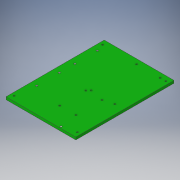
# Autodesk Inventor part: ModBoard-Bottom
Saved by Autodesk Inventor 2018 (Build 220112000, 112)
## iProperties
Created: 2017-12-22
Part Number: ModBoard-Bottom
Material: Generic
Document SubType Name: Modeling
Designer: jklei
Density: 1 g/cm^3
Appearance: Default
Author: jklei
Autodesk Inventor part; units mm, degrees
ref_plane "YZ Plane" through (0, 0, 0) normal (1, 0, 0) x (0, 1, 0)
ref_plane "XZ Plane" through (0, 0, 0) normal (0, 1, 0) x (-1, 0, 0)
ref_plane "XY Plane" through (0, 0, 0) normal (0, 0, 1) x (1, 0, 0)
sketch "Sketch1" plane through (0, 0, 0) normal (0, 1, 0) x (-1, 0, 0)
  line L0 (0, 0) -> (-171.45, 0)
  line L1 (-171.45, 0) -> (-171.45, -241.3)
  line L2 (-171.45, -241.3) -> (0, -241.3)
  line L3 (0, -241.3) -> (0, 0)
  dimension "d0" = 171.45
  dimension "d1" = 241.3
  constraints: 8 end point, 2 parallel, 1 horizontal, 1 perpendicular
  measures "d0" distance of L2.end L1.end
  measures "d1" distance of L1.end L0.end
extrude "Extrusion1" add sketch "Sketch1" along normal blind 6.35
sketch "Sketch2" plane through (0, 6.35, 0) normal (0, 1, 0) x (1, 0, 0)
  line L0 (0, 0) -> (8, 0)
  line L1 (0, 0) -> (171.45, 0) projected
  line L2 (8, 0) -> (8, 12)
  line L3 (171.45, 0) -> (163.45, 0)
  line L4 (163.45, 0) -> (163.45, 12)
  line L5 (171.45, 241.3) -> (0, 241.3) projected
  line L6 (0, 241.3) -> (8, 241.3)
  line L7 (8, 241.3) -> (8, 229.3)
  line L8 (171.45, 241.3) -> (163.45, 241.3)
  line L9 (163.45, 241.3) -> (163.45, 229.3)
  circle A0 centre (8, 229.3) radius 2.1
  circle A1 centre (163.45, 229.3) radius 2.1
  circle A2 centre (163.45, 12) radius 2.1
  circle A3 centre (8, 12) radius 2.1
  dimension "d4" = 8
  dimension "d5" = 12
  dimension "d6" = 8
  dimension "d7" = 12
  dimension "d8" = 8
  dimension "d9" = 12
  dimension "d10" = 8
  dimension "d11" = 12
  dimension "d12" = 4.2
  dimension "d13" = 4.2
  dimension "d14" = 4.2
  dimension "d15" = 4.2
  constraints: 16 end point, 4 centre point, 4 coincident, 4 perpendicular, 4 point on line
  measures "d4" distance of L0.start L0.end
  measures "d5" distance of L0.end L2.end
  measures "d6" distance of L1.end L3.end
  measures "d7" distance of L3.end L4.end
  measures "d8" distance of L5.end L6.end
  measures "d9" distance of L6.end L7.end
  measures "d10" distance of L5.start L8.end
  measures "d11" distance of L8.end L9.end
  measures "d12" diameter of A0
  measures "d13" diameter of A1
  measures "d14" diameter of A2
  measures "d15" diameter of A3
extrude "Extrusion2" cut sketch "Sketch2" against normal blind 25.4
sketch "Sketch3" plane through (0, 6.35, 0) normal (0, 1, 0) x (1, 0, 0)
  circle A0 centre (163.45, 12) radius 2.1 projected
  circle A1 centre (8, 229.3) radius 2.1 projected
  circle A2 centre (163.45, 229.3) radius 2.1 projected
  circle A3 centre (8, 12) radius 2.1 projected
  line L0 (0, 0) -> (171.45, 0) projected
  line L1 (171.45, 0) -> (171.45, 241.3) projected
  line L2 (171.45, 241.3) -> (0, 241.3) projected
  line L3 (0, 241.3) -> (0, 0) projected
  line L4 (163.45, 229.3) -> (149.45, 229.3)
  line L5 (149.45, 229.3) -> (91.45, 229.3)
  circle A4 centre (149.45, 229.3) radius 2.1
  circle A5 centre (91.45, 229.3) radius 2.1
  circle A6 centre (149.45, 118.048) radius 2.1
  circle A7 centre (91.45, 118.048) radius 2.1
  line L6 (171.45, 0) -> (125.095, 0)
  line L7 (0, 0) -> (171.45, 0) projected
  line L8 (125.095, 0) -> (125.095, 47.0154)
  circle A8 centre (125.095, 47.0154) radius 2.1
  line L9 (125.095, 47.0154) -> (85.095, 47.0154)
  circle A9 centre (85.095, 47.0154) radius 2.1
  line L10 (125.095, 47.0154) -> (125.095, 111.0234)
  line L11 (125.095, 111.0234) -> (85.095, 111.0234)
  circle A10 centre (85.095, 111.0234) radius 2.1
  circle A11 centre (125.095, 111.0234) radius 2.1
  line L12 (8, 229.3) -> (14.35, 229.3)
  line L13 (14.35, 229.3) -> (14.35, 210.25)
  circle A12 centre (14.35, 210.25) radius 2.1
  line L14 (14.35, 210.25) -> (14.35, 154.751)
  circle A13 centre (14.35, 154.751) radius 2.1
  line L15 (14.35, 154.751) -> (14.35, 116.651)
  circle A14 centre (14.35, 116.651) radius 2.1
  line L16 (14.35, 116.651) -> (14.35, 61.152)
  circle A15 centre (14.35, 61.152) radius 2.1
  dimension "d22" = 14
  dimension "d23" = 58
  dimension "d24" = 4.2
  dimension "d25" = 4.2
  dimension "d28" = 4.2
  dimension "d29" = 111.252
  dimension "d30" = 0
  dimension "d31" = 4.2
  dimension "d32" = 58
  dimension "d33" = 111.252
  dimension "d39" = 46.355
  dimension "d40" = 47.0154
  dimension "d41" = 4.2
  dimension "d42" = 40
  dimension "d43" = 4.2
  dimension "d44" = 64.008
  dimension "d45" = 4.2
  dimension "d46" = 4.2
  dimension "d51" = 6.35
  dimension "d52" = 4.2
  dimension "d53" = 19.05
  dimension "d54" = 55.499
  dimension "d55" = 4.2
  dimension "d56" = 38.1
  dimension "d57" = 4.2
  dimension "d58" = 55.499
  dimension "d59" = 4.2
  constraints: 24 end point, 12 centre point, 10 coincident, 4 vertical, 3 horizontal, 3 perpendicular, 2 point on line
  measures "d22" distance of L4.start L4.end
  measures "d23" distance of L4.end L5.end
  measures "d24" diameter of A4
  measures "d25" diameter of A5
  measures "d28" diameter of A6
  measures "d29" distance of A6.centre L4.end
  measures "d30" horizontal distance of A4.centre A6.centre
  measures "d31" diameter of A7
  measures "d32" distance of A6.centre A7.centre
  measures "d33" distance of A5.centre A7.centre
  measures "d39" distance of L0.end L6.end
  measures "d40" distance of L6.end L8.end
  measures "d41" diameter of A8
  measures "d42" distance of L9.start L9.end
  measures "d43" diameter of A9
  measures "d44" distance of L9.start L10.end
  measures "d45" diameter of A10
  measures "d46" diameter of A11
  measures "d51" distance of L12.start L12.end
  measures "d52" diameter of A12
  measures "d53" distance of L12.end L13.end
  measures "d54" distance of L14.start L14.end
  measures "d55" diameter of A13
  measures "d56" distance of L15.start L15.end
  measures "d57" diameter of A14
  measures "d58" distance of L16.start L16.end
  measures "d59" diameter of A15
extrude "Extrusion3" cut sketch "Sketch3" against normal blind 25.4 contours A4 L5 L4 | L4 L5 A4 | A5 | A6 | A7 | A8 L9 L8 | L8 L10 A8 | L9 A8 L10 | A9 | A11 L11 L10 | L10 L11 A11 | A10 | A12 L14 L13 | L13 L14 A12 | A13 L15 L14 | L14 L15 A13 | A14 L16 L15 | L15 L16 A14 | A15
sketch "Sketch4" plane through (0, 6.35, 0) normal (0, 1, 0) x (1, 0, 0)
  line L0 (0, 0) -> (171.45, 0) projected
  line L1 (171.45, 0) -> (131, 0)
  line L2 (131, 0) -> (131, 4.2)
  circle A0 centre (131, 4.2) radius 2.1
  dimension "d60" = 40.45
  dimension "d61" = 4.2
  dimension "d65" = 4.2
  constraints: 4 end point, 1 centre point, 1 coincident, 1 point on line, 1 vertical
  measures "d60" distance of L0.end L1.end
  measures "d61" distance of L1.end L2.end
  measures "d65" diameter of A0
extrude "Extrusion4" cut sketch "Sketch4" against normal blind 25.4
body "Solid1"
